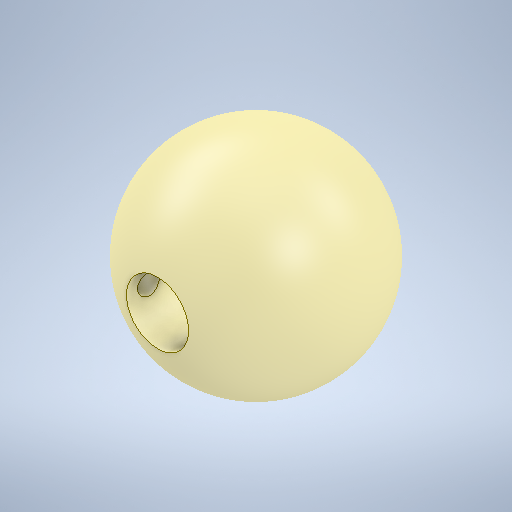
# Autodesk Inventor part: Esfera_0002_001
Saved by Autodesk Inventor 2025.2 (Build 292293000, 293)
## iProperties
Created: 2025-03-26
Part Number: Esfera_0002_001
Material: Náilon 6/6
Document SubType Name: Modeling
Designer: lucas
Density: 1.13 g/cm^3
Appearance: Náilon 6
Author: lucas
Autodesk Inventor part; units mm, degrees
ref_plane "YZ Plane" through (0, 0, 0) normal (1, 0, 0) x (0, 1, 0)
ref_plane "XZ Plane" through (0, 0, 0) normal (0, 1, 0) x (-1, 0, 0)
ref_plane "XY Plane" through (0, 0, 0) normal (0, 0, 1) x (1, 0, 0)
sketch "Esboço1" plane through (0, 0, 0) normal (0, 0, 1) x (1, 0, 0)
  circle A0 centre (0, 0) radius 5 construction
  arc A1 (0, -5) -> (0, 5) centre (0, 0) ccw
  arc A2 (0, -3) -> (0, 3) centre (0, 0) ccw
  line L0 (0, 5) -> (0, -5)
  point P0 (3, 0)
  point P1 (5, 0)
  point P2 (0, 3)
  dimension "d0" = 10
  dimension "d2" = 3
  constraints: 8 point on circle, 5 vertical alignment, 3 centre point, 3 horizontal alignment, 2 coincident, 2 end point, 1 concentric, 1 midpoint, 1 vertical
  measures "d0" diameter of A0
  measures "d2" radius of A2
revolve "Revolução1" add sketch "Esboço1" angle 360 about axis through (0, 5, 0) along (0, -1, 0) contours L0 A2 A1
sketch "Esboço2" plane through (0, 0, 0) normal (0, 0, 1) x (1, 0, 0)
  circle A0 centre (4, 0) radius 0.5
  line L0 (0, 5) -> (0, -5)
  point P0 (0, 0)
  point P1 (0, 0)
  dimension "d4" = 1
  dimension "d5" = 4
  dimension "d6" = 10
  constraints: 2 coincident, 2 end point, 1 centre point, 1 horizontal alignment, 1 midpoint, 1 vertical
  measures "d4" diameter of A0
  measures "d5" distance of point (0, 0) A0.centre
  measures "d6" distance of L0.start L0.end
revolve "Revolução2" cut sketch "Esboço2" angle 360 about axis through (0, 5, 0) along (0, 1, 0)
sketch "Esboço4" plane through (0, 0, 0) normal (0, 0, 1) x (1, 0, 0)
  circle A0 centre (0, 0) radius 1.5
  dimension "d10" = 3
  constraints: 1 centre point, 1 coincident
  measures "d10" diameter of A0
extrude "Extrusão1" cut sketch "Esboço4" along normal through all both and the other way through all
